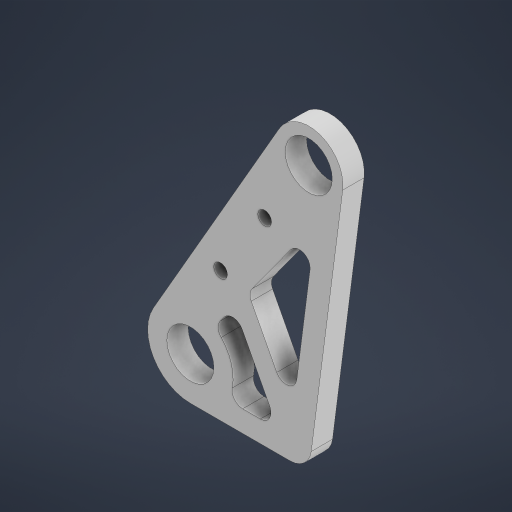
# Autodesk Inventor part: Intake_FourBar_Plate
Saved by Autodesk Inventor 2023 (Build 270158000, 158)
## iProperties
Created: 2023-03-17
Part Number: Intake_FourBar_Plate
Material: Generic
Document SubType Name: Modeling
Designer: kelle
Density: 1 g/cm^3
Appearance: Default
Author: kelle
Autodesk Inventor part; units mm, degrees
ref_plane "YZ Plane" through (0, 0, 0) normal (1, 0, 0) x (0, 1, 0)
ref_plane "XZ Plane" through (0, 0, 0) normal (0, 1, 0) x (-1, 0, 0)
ref_plane "XY Plane" through (0, 0, 0) normal (0, 0, 1) x (1, 0, 0)
sketch "Sketch1" plane through (0, 0, 0) normal (0, 0, 1) x (1, 0, 0)
  circle A0 centre (0, 0) radius 7
  line L0 (0, 0) -> (0, -11.43) construction
  line L1 (0, -11.43) -> (-50.8, -11.43) construction
  circle A1 centre (-50.8, -11.43) radius 7
  line L2 (0, -11.43) -> (0, -24.13) construction
  line L3 (-50.8, -11.43) -> (-50.8, -24.13) construction
  line L4 (0, -24.13) -> (-101.6, -24.13) construction
  line L5 (-101.6, -24.13) -> (-101.6, -125.73) construction
  line L6 (0, -24.13) -> (12.7, -24.13) construction
  line L7 (-101.6, -125.73) -> (-35.3, -24.13) construction
  line L8 (-101.6, -125.73) -> (15.6852, -125.73) construction
  line L9 (-35.3, -24.13) -> (-117.1955, 29.3117) construction
  line L10 (-117.1955, 29.3117) -> (-143.4272, -10.8866) construction
  line L11 (-123.0577, 33.1371) -> (-149.2895, -7.0611) construction
  line L12 (-137.565, -14.712) -> (-111.3333, 25.4862) construction
  arc A2 (-111.3333, 25.4862) -> (-123.0577, 33.1371) centre (-117.1955, 29.3117) ccw construction
  arc A3 (-149.2895, -7.0611) -> (-137.565, -14.712) centre (-143.4272, -10.8866) ccw construction
  circle A4 centre (-117.1955, 29.3117) radius 12.7 construction
  circle A5 centre (0, 0) radius 120.8055 construction
  circle A6 centre (-50.8, -11.43) radius 92.6288 construction
  line L13 (-101.6, -125.73) -> (-152.4, -125.73) construction
  line L14 (-152.4, -125.73) -> (-152.4, -87.63) construction
  circle A7 centre (-152.4, -87.63) radius 38.1
  line L15 (-152.4, -87.63) -> (-152.4, -49.53) construction
  line L16 (-152.4, -49.53) -> (-152.4, -36.83) construction
  circle A8 centre (-152.4, -36.83) radius 12.7 construction
  circle A9 centre (-117.1955, 29.3117) radius 10.16
  circle A10 centre (-152.4, -36.83) radius 12.7
  line L17 (-163.4022, -30.4863) -> (-125.9972, 34.3866)
  line L18 (-152.4, -49.53) -> (-117.1955, -49.53)
  circle A11 centre (-130.3114, 9.2125) radius 2.05
  circle A12 centre (-143.4272, -10.8866) radius 2.05
  circle A13 centre (-117.1955, 29.3117) radius 7
  circle A14 centre (-152.4, -36.83) radius 7
  line L19 (-117.1955, -49.53) -> (-107.1202, 28.0024)
  point P0 (-152.4, -49.53)
  dimension "d0" = 14
  dimension "d1" = 11.43
  dimension "d2" = 50.8
  dimension "d3" = 14
  dimension "d4" = 12.7
  dimension "d5" = 12.7
  dimension "d6" = 101.6
  dimension "d7" = 101.6
  dimension "d8" = 12.7
  dimension "d9" = 48
  dimension "d14" = 97.79
  dimension "d15" = 90
  dimension "d16" = 48
  dimension "d17" = 14
  dimension "d18" = 25.4
  dimension "d19" = 50.8
  dimension "d20" = 38.1
  dimension "d21" = 12.7
  dimension "d22" = 20.32
  dimension "d24" = 4.1
  dimension "d25" = 4.1
  dimension "d26" = 14
  constraints: 42 end point, 12 centre point, 12 coincident, 10 point on circle, 7 tangent, 7 vertical, 6 horizontal, 4 point on line, 2 parallel, 1 concentric, 1 midpoint, 1 vertical alignment, 9 other
  measures "d0" diameter of A0
  measures "d1" distance of L0.start L0.end
  measures "d2" distance of L0.end L1.end
  measures "d3" diameter of A1
  measures "d4" distance of L0.end L2.end
  measures "d5" distance of L3.start L3.end
  measures "d6" distance of L2.end L4.end
  measures "d7" distance of L4.end L5.end
  measures "d8" distance of L2.end L6.end
  measures "d9" distance of L6.end L7.end
  measures "d14" distance of L7.end L9.end
  measures "d15" angle of L7 L9
  measures "d16" distance of L9.end L10.end
  measures "d17" diameter of A3
  measures "d18" diameter of A4
  measures "d19" distance of L5.end L13.end
  measures "d20" distance of L13.end L14.end
  measures "d21" distance of L15.end L16.end
  measures "d22" diameter of A9
  measures "d24" diameter of A11
  measures "d25" diameter of A12
  measures "d26" diameter of A14
extrude "Extrusion1" add sketch "Sketch1" along normal blind 6.35 contours A10 | A10 L17 A9 L19 L18 | A9
fillet "Fillet1" radius 6.35 1 edges at (-117.1955, -49.53, 3.175)
sketch "Sketch2" plane through (0, 0, 6.35) normal (0, 0, 1) x (1, 0, 0)
  circle A0 centre (-152.4, -36.83) radius 7 construction
  circle A1 centre (-152.4, -36.83) radius 12.7
  circle A2 centre (-117.1955, 29.3117) radius 7 construction
  circle A3 centre (-117.1955, 29.3117) radius 10.16
  line L0 (-125.9972, 34.3866) -> (-163.4022, -30.4863) construction
  arc A4 (-122.7737, -49.53) -> (-116.4767, -43.9983) centre (-122.7737, -43.18) ccw construction
  line L1 (-152.4, -49.53) -> (-122.7737, -49.53) construction
  line L2 (-116.4767, -43.9983) -> (-107.1202, 28.0024) construction
  line L3 (-122.7737, -43.18) -> (-114.631, 19.4806)
  line L4 (-122.7737, -43.18) -> (-149.4542, -43.18)
  circle A5 centre (-143.4272, -10.8866) radius 2.05 projected
  line L5 (-143.4272, -10.8866) -> (-130.3114, 7.1625) construction
  circle A6 centre (-130.3114, 9.2125) radius 2.05 projected
  line L6 (-145.2764, -26.316) -> (-115.2046, 15.0667)
  line L7 (-136.4387, 11.6152) -> (-149.5546, -6.434)
  arc A7 (-149.5546, -6.434) -> (-137.2998, -15.3392) centre (-143.4272, -10.8866) ccw
  arc A8 (-124.184, 2.7099) -> (-136.4387, 11.6152) centre (-130.3114, 7.1625) ccw
  line L8 (-122.7737, -43.18) -> (-137.2998, -15.3392) construction
  line L9 (-119.9588, -41.7113) -> (-134.485, -13.8705)
  line L10 (-140.1147, -16.8079) -> (-125.5886, -44.6487)
  arc A9 (-125.5886, -44.6487) -> (-119.9588, -41.7113) centre (-122.7737, -43.18) ccw
  arc A10 (-134.485, -13.8705) -> (-140.1147, -16.8079) centre (-137.2998, -15.3392) ccw
  point P0 (0, 0)
  point P1 (-136.8693, -1.862)
  point P2 (-130.0368, -29.2596)
  point P3 (-135.4334, -12.7707)
  point P4 (-122.0596, -37.6849)
  point P5 (-126.3549, -43.18)
  point P6 (-139.3843, -18.2077)
  point P7 (-141.4015, -43.18)
  dimension "d30" = 6.35
  constraints: 20 end point, 10 point on circle, 9 tangent, 6 centre point, 3 parallel, 3 point on line, 2 coincident, 2 midpoint, 1 horizontal, 1 vertical alignment, 3 other
  measures "d30" diameter of A10
extrude "Extrusion2" cut sketch "Sketch2" against normal through all contours A1 L6 L10 L4 | L6 L3 L9 A10
fillet "Fillet2" radius 3.175 7 edges at (-115.2046, 15.0667, 3.175) (-122.0596, -37.6849, 3.175) (-135.4334, -12.7707, 3.175) (-139.3843, -18.2077, 3.175) (-126.3549, -43.18, 3.175) (-141.4015, -43.18, 3.175) (-145.2764, -26.316, 3.175)
body "Solid1"
